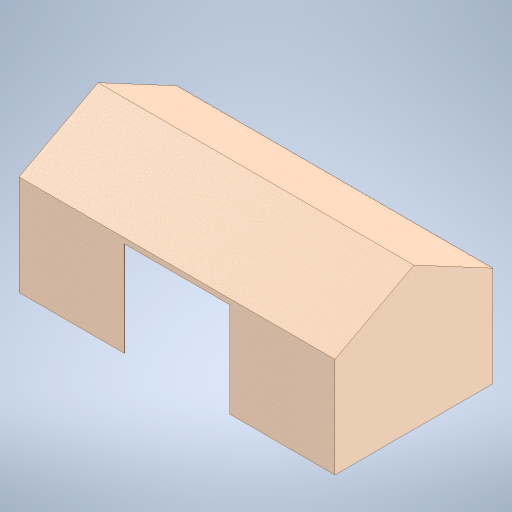
# Autodesk Inventor part: BungaCamp-CostcoCarport
Saved by Autodesk Inventor 2023 (Build 270158000, 158)
## iProperties
Created: 2024-07-15
Part Number: BungaCamp-CostcoCarport
Material: Generic
Document SubType Name: Modeling
Designer: incep
Density: 1 g/cm^3
Appearance: Default
Author: incep
Autodesk Inventor part; units mm, degrees
ref_plane "YZ Plane" through (0, 0, 0) normal (1, 0, 0) x (0, 1, 0)
ref_plane "XZ Plane" through (0, 0, 0) normal (0, 1, 0) x (-1, 0, 0)
ref_plane "XY Plane" through (0, 0, 0) normal (0, 0, 1) x (1, 0, 0)
sketch "Sketch1" plane through (0, 0, 0) normal (0, 1, 0) x (-1, 0, 0)
  line L0 (3000, -1500) -> (-3000, -1500)
  line L1 (-3000, -1500) -> (-3000, 1500)
  line L2 (-3000, 1500) -> (3000, 1500)
  line L3 (3000, 1500) -> (3000, -1500)
  line L4 (2990, 1490) -> (-2990, 1490)
  line L5 (-2990, 1490) -> (-2990, -1490)
  line L6 (-2990, -1490) -> (2990, -1490)
  line L7 (2990, -1490) -> (2990, 1490)
  point P0 (0, 0)
  point P1 (-3000, 0)
  point P2 (0, -1500)
  dimension "d0" = 3000
  dimension "d1" = 6000
  dimension "d2" = 10
  constraints: 16 end point, 4 parallel, 2 midpoint, 2 perpendicular, 1 horizontal, 1 horizontal alignment, 1 vertical alignment, 3 other
  measures "d0" distance of L2.end L0.start
  measures "d1" distance of L0.start L0.end
  measures "d2" distance between parallel lines of L2 L4
extrude "Extrusion1" add sketch "Sketch1" along normal blind 1900
sketch "Sketch2" plane through (3000, 0, 1500) normal (1, 0, 0) x (0, 0, -1)
  line L0 (0, 1900) -> (3000, 1900) projected
  line L1 (0, 0) -> (0, 1900) projected
  line L2 (0, 1900) -> (1500, 2700)
  line L3 (3000, 0) -> (3000, 1900) projected
  line L4 (1500, 2700) -> (3000, 1900)
  line L5 (4.7059, 1891.1765) -> (1500, 2688.6667)
  line L6 (1500, 2688.6667) -> (2995.2941, 1891.1765)
  point P0 (1500, 0)
  point P1 (2990, 1900)
  point P2 (1500, 1900)
  point P3 (21.25, 1900)
  point P4 (2978.75, 1900)
  dimension "d5" = 1700
  dimension "d6" = 10
  constraints: 8 end point, 1 midpoint, 1 vertical alignment, 1 other
  measures "d5" distance of L0.start L2.end
  measures "d6" distance between parallel lines of L2 L5
extrude "Extrusion2" add sketch "Sketch2" against normal up to surface (6000 mm away) contours L2 L4 L0 L6 L5
sketch "Sketch3" plane through (-3000, 0, -1500) normal (-1, 0, 0) x (0, 0, 1)
  line L0 (21.25, 1900) -> (2978.75, 1900) projected
  line L1 (1500, 2688.6667) -> (21.25, 1900) projected
  line L2 (2978.75, 1900) -> (1500, 2688.6667) projected
  point P0 (1500, 0)
extrude "Extrusion3" add sketch "Sketch3" against normal blind 10
sketch "Sketch4" plane through (3000, 0, 1500) normal (1, 0, 0) x (0, 0, -1)
  line L0 (21.25, 1900) -> (1500, 2688.6667) projected
  line L1 (21.25, 1900) -> (2978.75, 1900) projected
  line L2 (1500, 2688.6667) -> (2978.75, 1900) projected
  point P0 (1500, 0)
extrude "Extrusion4" add sketch "Sketch4" against normal blind 10
sketch "Sketch5" plane through (-3000, 0, 1500) normal (0, 0, 1) x (1, 0, 0)
  line L0 (2000, 1800) -> (4000, 1800)
  line L1 (4000, 1800) -> (4000, 0)
  line L2 (4000, 0) -> (2000, 0)
  line L3 (2000, 0) -> (2000, 1800)
  line L4 (0, 0) -> (6000, 0) projected
  line L5 (0, 1900) -> (6000, 1900) projected
  point P0 (3000, 0)
  point P1 (3000, 0)
  point P2 (3000, 0)
  dimension "d13" = 100
  dimension "d14" = 2000
  constraints: 8 end point, 2 midpoint, 2 parallel, 1 coincident, 1 collinear, 1 horizontal, 1 perpendicular
  measures "d13" distance between parallel lines of L5 L0
  measures "d14" distance between parallel lines of L1 L3
extrude "Extrusion5" cut sketch "Sketch5" against normal up to surface (10 mm away)
body "Solid1"
